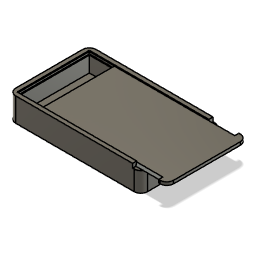
scissors_box (Autodesk Fusion 360 design; units mm, degrees)
Autodesk Fusion 360 part; units mm, degrees
sketch "base" plane through (0, 0, 0) normal (0, 1, 0) x (1, 0, 0)
  line L0 (0, 0) -> (120, 0)
  line L1 (120, 0) -> (120, -70)
  line L2 (120, -70) -> (0, -70)
  line L3 (0, -70) -> (0, 0)
  line L4 (124, -74) -> (-4, -74)
  line L5 (-4, -74) -> (-4, 4)
  line L6 (-4, 4) -> (124, 4)
  line L7 (124, 4) -> (124, -74)
  dimension "d1" = 120
  dimension "d2" = 70
  dimension "d3" = -4
  constraint horizontal L0
  constraint vertical L1
  constraint horizontal L2
  constraint vertical L3
  constraint coincident L0.start L3.end
  measures "d1" distance of L0.start L0.end
  measures "d2" distance of L0.start L2.end
extrude "Extrude1" add sketch "base" along normal blind 4 contours L0 L1 L2 L3 makes body 1
extrude "Extrude2" add sketch "base" along normal blind 19 bodies 1
sketch "Sketch2" plane through (0, 19, 0) normal (0, 1, 0) x (-1, 0, 0)
  line L0 (-120, 70) -> (0, 70)
  line L1 (0, 70) -> (0, 0)
  line L2 (0, 0) -> (-120, 0)
  line L3 (-120, 0) -> (-120, 70)
  line L4 (-124, -4) -> (4, -4)
  line L5 (4, -4) -> (4, 74)
  line L6 (4, 74) -> (-124, 74)
  line L7 (-124, 74) -> (-124, -4)
  line L8 (-120, 0) -> (-120, 10)
  line L9 (-120, 10) -> (-124, 10)
  line L10 (-120, 0) -> (-124, 0)
  line L11 (-120, 0) -> (-120, 3)
  line L12 (-120, 3) -> (-116, 3)
  line L13 (-116, 3) -> (-116, 0)
  line L14 (-124, 35) -> (4, 35)
  line L15 (-120, 67) -> (-116, 67)
  line L16 (-116, 67) -> (-116, 70)
  line L17 (-120, 70) -> (-120, 60)
  line L18 (-120, 60) -> (-124, 60)
  line L19 (-120, 70) -> (-124, 70)
  line L20 (-116, 0) -> (-116, -4)
  line L21 (-116, 70) -> (-116, 74)
  dimension "d8" = 10
  dimension "d9" = 3
  dimension "d10" = 4
  constraint coincident L2.end L3.start
  constraint perpendicular L2 L8
  constraint coincident L7 L9.end
  constraint perpendicular L7 L9
  constraint coincident L7 L10.end
  constraint perpendicular L7 L10
  constraint perpendicular L2 L11
  constraint perpendicular L8 L12
  constraint coincident L2 L13.end
  constraint perpendicular L2 L13
  constraint midpoint L7 L14.start
  constraint midpoint L5 L14.end
  constraint symmetric L2.end L14 L0.start
  constraint symmetric L8.end L14 L17.end
  constraint symmetric L9.end L14 L18.end
  constraint symmetric L10.end L14 L19.end
  constraint symmetric L11.end L14 L15.start
  constraint symmetric L12.end L14 L15.end
  constraint symmetric L13.end L14 L16.end
  constraint coincident L4 L20.end
  constraint perpendicular L4 L20
  constraint coincident L6 L21.end
  constraint perpendicular L6 L21
  measures "d8" distance of L2.end L8.end
  measures "d9" distance of L2.end L11.end
  measures "d10" distance of L11.end L12.end
extrude "Extrude4" add sketch "Sketch2" along normal blind 4 contours L0 L1 L5 L6 L14 L21 | L1 L2 L4 L5 L14 L20 bodies 1
sketch "Sketch3" plane through (116, 0, 0) normal (1, 0, 0) x (0, 0, -1)
  line L0 (-74, 19) -> (-70, 19)
  line L1 (-70, 19) -> (-70, 23)
  line L2 (-70, 23) -> (-74, 23)
  line L3 (-74, 23) -> (-74, 19)
  line L4 (-70, 23) -> (-70, 22)
  line L5 (-72, 19) -> (-71, 19)
  line L6 (-71, 19) -> (-70, 22)
  line L7 (-71, 22) -> (-71, 19)
  line L8 (-70, 23) -> (0, 23)
  line L9 (-35, 23) -> (-35, 6.2814)
  line L10 (1, 19) -> (0, 22)
  line L11 (1, 22) -> (1, 19)
  line L12 (0, 23) -> (0, 22)
  line L13 (0, 19) -> (0, 23)
  line L14 (4, 19) -> (0, 19)
  line L15 (-71, 22) -> (-70, 22)
  line L16 (1, 22) -> (0, 22)
  dimension "d15" = 1
  dimension "d16" = 1
  constraint coincident L1.end L2.start
  constraint perpendicular L2 L4
  constraint coincident L0.start L5.start
  constraint midpoint L0 L5.end
  constraint midpoint L8 L9.start
  constraint perpendicular L8 L9
  constraint symmetric L0.start L9 L14.start
  constraint symmetric L0.end L9 L13.start
  constraint symmetric L1.end L9 L8.end
  constraint symmetric L4.end L9 L10.end
  constraint symmetric L5.end L9 L10.start
  constraint symmetric L7.start L9 L11.start
  measures "d15" distance of L1.end L4.end
  measures "d16" distance of L5.start L5.end
fillet "Fillet2" radius 6.5 4 edges at (-4, 11.5, 74) (124, 9.5, 74) (124, 9.5, -4) (-4, 11.5, -4) on bodies 1
ref_plane "WorkPlane1" through (120, 19, 35) normal (0, 1, 0) x (0, 0, 1)
sweep "Sweep3" cut profiles "Sketch3" along 3 edges at (58, 23, 70) (0, 23, 35) (58, 23, 0) section 1 contours L0 L1 L6 | L6 L7 L15 on bodies 1 bodies 1
sweep "Sweep4" add profiles "Sketch3" along 1 edges at (58, 23, 70) section 1 contours L6 L7 L15 on bodies 1 bodies 1
extrude "Extrude5" add 1 faces at (0, 21, 70.6667) along direction (-1, 0, 0) blind 1.5 on bodies 1 bodies 1
sweep "Sweep5" add profiles "Sketch3" along 1 edges at (57.5, 19, -1) section 1 contours L10 L11 L16 on bodies 1 bodies 1
sketch "Sketch6" plane through (0, 19, 0) normal (0, 1, 0) x (1, 0, 0)
  line L0 (227.1637, -44.8349) -> (102.4637, -44.8349)
  line L1 (102.4637, -44.8349) -> (102.4637, 26.8651)
  line L2 (102.4637, 26.8651) -> (227.1637, 26.8651)
  line L3 (227.1637, 26.8651) -> (227.1637, -44.8349)
  dimension "d58" = 124.7
  dimension "d59" = 71.7
  constraint horizontal L0
  constraint vertical L1
  constraint horizontal L2
  constraint vertical L3
  measures "d58" distance of L0.start L0.end
  measures "d59" distance of L0.start L2.end
extrude "Extrude6" add sketch "Sketch6" along normal blind 3 separate body makes body 2
move_body "Move1" bodies 2 to x (1, 0, 0) y (0, 1, 0) z (0, 0, 1) at (54.343, -3.051, -4.5628)
sketch "Sketch7" plane through (281.5067, 0, 0) normal (1, 0, 0) x (0, 0, -1)
  line L0 (-40.2721, 15.949) -> (31.4279, 15.949)
  line L1 (31.4279, 15.949) -> (31.4279, 18.949)
  line L2 (31.4279, 18.949) -> (-40.2721, 18.949)
  line L3 (-40.2721, 18.949) -> (-40.2721, 15.949)
  line L4 (-40.2721, 15.949) -> (-39.2721, 15.949)
  line L5 (-40.2721, 18.949) -> (-39.2721, 18.949)
  line L6 (-39.2721, 18.949) -> (-40.2721, 15.949)
  line L7 (-4.4221, 18.949) -> (-4.4221, 15.949)
  line L8 (30.4279, 18.949) -> (31.4279, 15.949)
  line L9 (31.4279, 18.949) -> (30.4279, 18.949)
  line L10 (31.4279, 15.949) -> (30.4279, 15.949)
  dimension "d62" = 1
  dimension "d63" = 1
  constraint coincident L0.start L3.end
  constraint coincident L0 L4.end
  constraint coincident L2.end L3.start
  constraint perpendicular L3 L5
  constraint midpoint L2 L7.start
  constraint midpoint L0 L7.end
  constraint symmetric L0.start L7 L0.end
  constraint symmetric L4.end L7 L10.end
  constraint symmetric L2.end L7 L1.end
  constraint symmetric L5.end L7 L8.start
  measures "d62" distance of L0.start L4.end
  measures "d63" distance of L2.end L5.end
extrude "Extrude7" cut sketch "Sketch7" against normal blind 135 contours L2 L3 L5 L6 | L1 L2 L8 L9 bodies 2
move_body "Move2" bodies 2 to x (1, 0, 0) y (0, 1, 0) z (0, 0, 1) at (0, 0, 30.5)
move_body "Move3" bodies 2 to x (1, 0, 0) y (0, 1, 0) z (0, 0, 1) at (0, 3, 0)
move_body "Move4" bodies 2 to x (1, 0, 0) y (0, 1, 0) z (0, 0, 1) at (-76, 0, 0)
move_body "Move5" bodies 2 to x (1, 0, 0) y (0, 1, 0) z (0, 0, 1) at (-81.5, 0, 0)
move_body "Move6" bodies 2 to x (1, 0, 0) y (0, 1, 0) z (0, 0, 1) at (25, 0, 0)
sketch "Sketch10" plane through (0, 21.949, 0) normal (0, 1, 0) x (-1, 0, 0)
  line L0 (-24.3067, 69.7721) -> (-149.0067, 69.7721)
  line L1 (-149.0067, 69.7721) -> (-149.0067, 0.0721)
  line L2 (-149.0067, 0.0721) -> (-24.3067, 0.0721)
  line L3 (-24.3067, 0.0721) -> (-24.3067, 69.7721)
  line L4 (-24.3067, -0.9279) -> (-149.0067, -0.9279)
  line L5 (-149.0067, -0.9279) -> (-149.0067, 0.0721)
  line L6 (-149.0067, 0.0721) -> (-141.1067, 0.0721)
  line L7 (-141.1067, 0.0721) -> (-141.1067, -0.9279)
  line L8 (-149.0067, 34.9221) -> (-119.7376, 34.9221)
  line L9 (-24.3067, 70.7721) -> (-149.0067, 70.7721)
  line L10 (-149.0067, 69.7721) -> (-141.1067, 69.7721)
  line L11 (-141.1067, 69.7721) -> (-141.1067, 70.7721)
  line L12 (-149.0067, 70.7721) -> (-149.0067, 69.7721)
  dimension "d69" = 7.9
  constraint coincident L1.end L2.start
  constraint perpendicular L5 L6
  constraint coincident L4 L7.end
  constraint perpendicular L4 L7
  constraint midpoint L1 L8.start
  constraint perpendicular L1 L8
  constraint symmetric L4.start L8 L9.start
  constraint symmetric L4.end L8 L9.end
  constraint symmetric L1.end L8 L0.end
  constraint symmetric L6.end L8 L10.end
  constraint symmetric L7.end L8 L11.end
  measures "d69" distance of L1.end L6.end
extrude "Extrude8" cut sketch "Sketch10" against normal blind 10 contours L0 L9 L10 L11 L12 | L2 L4 L5 L6 L7 bodies 2
move_body "Move7" bodies 2 to x (1, 0, 0) y (0, 1, 0) z (0, 0, 1) at (-25, 0, 0)
sketch "Sketch11" plane through (0, 21.949, 0) normal (0, 1, 0) x (-1, 0, 0)
  line L0 (0.6933, 69.7721) -> (-116.1067, 69.7721)
  line L1 (-116.1067, 69.7721) -> (-124.0067, 69.7721)
  line L2 (-124.0067, 69.7721) -> (-124.0067, 0.0721)
  line L3 (-124.0067, 0.0721) -> (-116.1067, 0.0721)
  line L4 (-116.1067, 0.0721) -> (0.6933, 0.0721)
  line L5 (0.6933, 0.0721) -> (0.6933, 69.7721)
  arc A0 (-124, 2.5) -> (-117.5, -4) centre (-117.5, 2.5) ccw
  line L6 (-117.5, -4) -> (-116, -4)
  line L7 (-116.1067, 0.0721) -> (-116.1067, -4)
  line L8 (-124, 2.5) -> (-116.1067, 0.0721)
  arc A1 (-125, 2.5) -> (-117.5, -5) centre (-117.5, 2.5) ccw
  line L9 (-117.5, -5) -> (-116, -5)
  line L10 (-124, 2.5) -> (-125, 2.5)
  line L11 (-116.1067, -4) -> (-116, -5)
  line L12 (-124.0067, 34.9221) -> (-86.6091, 34.9221)
  line L13 (-124.0067, 69.7721) -> (-116.1067, 69.7721)
  line L14 (-116.1067, 73.8443) -> (-116, 74.8443)
  line L15 (-116.1067, 69.7721) -> (-116.1067, 73.8443)
  line L16 (-124, 67.3443) -> (-116.1067, 69.7721)
  line L17 (-117.5, 73.8443) -> (-116, 73.8443)
  line L18 (-124, 67.3443) -> (-125, 67.3443)
  arc A2 (-117.5, 73.8443) -> (-124, 67.3443) centre (-117.5, 67.3443) ccw
  arc A3 (-117.5, 74.8443) -> (-125, 67.3443) centre (-117.5, 67.3443) ccw
  line L19 (-117.5, 74.8443) -> (-116, 74.8443)
  dimension "d72" = 1
  constraint coincident L3.end L4.start
  constraint coincident L6 L7.end
  constraint perpendicular L6 L7
  constraint coincident A0.start L8.start
  constraint horizontal L10
  constraint midpoint L2 L12.start
  constraint perpendicular L2 L12
  constraint symmetric L2.end L12 L1.end
  constraint symmetric L3.end L12 L0.end
  constraint symmetric A0.start L12 L16.start
  constraint symmetric A0.end L12 L17.start
  constraint symmetric A0 L12 A2
  constraint symmetric L6.end L12 L17.end
  constraint symmetric L7.end L12 L14.start
  constraint symmetric A1.end L12 A3.start
  constraint symmetric A1.start L12 L18.end
  constraint symmetric A1 L12 A3
  constraint symmetric L9.end L12 L14.end
extrude "Extrude9" add sketch "Sketch11" against normal blind 3 separate body contours L1 L13 L16 A2 | L1 L13 L15 L17 A2 | L3 A0 L6 L7 | L3 A0 L8 makes body 3 at (116.5711, 18.949, -2.6426) makes body 4 at (116.5711, 21.949, 72.4869)
extrude "Extrude10" cut sketch "Sketch11" against normal blind 3 contours L1 L2 L13 L18 A2 | L1 L2 L13 L14 L17 L18 A2 A3 L19 | L2 L3 A0 L6 A1 L9 L10 L11 | L2 L3 A0 L10 bodies 1 2
combine "Combine1" operation add target body 2 tool bodies 3 4
sketch "Sketch12" plane through (0, 18.949, 0) normal (0, -1, 0) x (1, 0, 0)
  line L0 (116.1067, 70.7721) -> (-0.6933, 70.7721)
  line L1 (-0.6933, 70.7721) -> (-0.6933, -0.9279)
  line L2 (-0.6933, -0.9279) -> (116.1067, -0.9279)
  line L3 (116.1067, -0.9279) -> (116.1067, -4)
  line L4 (116.1067, -4) -> (117.5, -4)
  arc A0 (117.5, -4) -> (124, 2.5) centre (117.5, 2.5) ccw
  line L5 (124, 2.5) -> (124.0067, 2.5)
  line L6 (124.0067, 2.5) -> (124.0067, 67.3443)
  line L7 (124.0067, 67.3443) -> (124, 67.3443)
  arc A1 (124, 67.3443) -> (117.5, 73.8443) centre (117.5, 67.3443) ccw
  line L8 (117.5, 73.8443) -> (116.1067, 73.8443)
  line L9 (116.1067, 73.8443) -> (116.1067, 70.7721)
  line L10 (120, 0) -> (120, 70)
  line L11 (0, 0) -> (120, 0)
  line L12 (120, 70) -> (0, 70)
  line L13 (116.1067, -0.9279) -> (116.1067, 70.7721)
  line L14 (116.1067, 34.9221) -> (95.1099, 34.9221)
  line L15 (116.1067, 34.9221) -> (116.1067, 30.9221)
  line L16 (116.1067, 30.9221) -> (119.1067, 30.9221)
  line L17 (119.1067, 30.9221) -> (106.1067, 30.9221)
  line L18 (106.1067, 30.9221) -> (106.1067, 34.9221)
  line L19 (106.1067, 34.9221) -> (116.1067, 34.9221)
  line L20 (116.1067, 34.9221) -> (119.1067, 34.9221)
  line L21 (119.1067, 34.9221) -> (119.1067, 30.9221)
  line L22 (116.1067, 34.9221) -> (119.1067, 34.9221)
  line L23 (116.1067, 34.9221) -> (116.1067, 38.9221)
  line L24 (106.1067, 34.9221) -> (116.1067, 34.9221)
  line L25 (119.1067, 34.9221) -> (119.1067, 38.9221)
  line L26 (106.1067, 38.9221) -> (106.1067, 34.9221)
  line L27 (119.1067, 38.9221) -> (106.1067, 38.9221)
  line L28 (116.1067, 38.9221) -> (119.1067, 38.9221)
  dimension "d77" = 4
  dimension "d78" = 3
  dimension "d79" = 13
  constraint coincident L2.end L3.start
  constraint coincident L0.start L9.end
  constraint midpoint L13 L14.start
  constraint perpendicular L13 L14
  constraint perpendicular L14 L15
  constraint perpendicular L10 L16
  constraint perpendicular L13 L17
  constraint coincident L14 L18.end
  constraint perpendicular L14 L18
  constraint perpendicular L15 L20
  constraint perpendicular L17 L21
  constraint symmetric L15.start L14 L19.end
  constraint symmetric L14 L15.end L23.end
  constraint symmetric L14 L16.end L25.end
  constraint symmetric L14 L17.end L26.start
  constraint symmetric L14 L18.end L19.start
  constraint symmetric L14 L20.end L21.start
  measures "d77" distance of L14.start L15.end
  measures "d78" distance of L15.end L16.end
  measures "d79" distance of L16.end L17.end
move_body "Move8" bodies 1 to x (1, 0, 0) y (0, 1, 0) z (0, 0, 1) at (-25, 0, 0)
extrude "Extrude11" add sketch "Sketch12" along normal blind 2 contours L13 L20 L22 L23 L25 L27 L28 | L13 L14 L19 L23 L24 L26 L27 | L13 L15 L16 L17 L20 L21 L22 | L13 L14 L15 L17 L18 L19 L24 bodies 2
sketch "Sketch13" plane through (0, 0, 38.9221) normal (0, 0, 1) x (1, 0, 0)
  line L0 (119.1067, 18.949) -> (106.1067, 18.949)
  line L1 (106.1067, 18.949) -> (106.1067, 16.949)
  line L2 (106.1067, 16.949) -> (119.1067, 16.949)
  line L3 (119.1067, 16.949) -> (119.1067, 18.949)
  line L4 (119.1067, 18.949) -> (109.1067, 18.949)
  line L5 (119.1067, 16.949) -> (109.1067, 18.949)
  dimension "d82" = 10
  constraint coincident L0.start L3.end
  constraint perpendicular L3 L4
  constraint coincident L2.end L3.start
  measures "d82" distance of L0.start L4.end
extrude "Extrude12" cut sketch "Sketch13" against normal blind 14 contours L0 L1 L2 L5 bodies 2
equation "d6 = 15 mm + 4 mm"
equation "d59 = 72 mm - 0.3 mm"
named bodies: "box", "lid"
